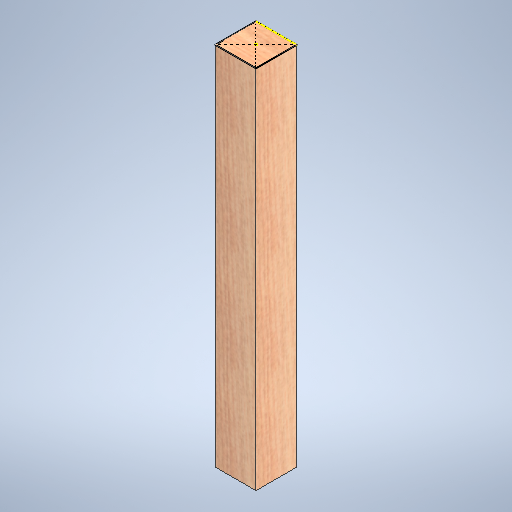
# Autodesk Inventor part: 4x4x36
Saved by Autodesk Inventor 2025 (Build 290162000, 162)
## iProperties
Created: 2024-06-05
Part Number: 4x4x36
Material: Wood (Birch)
Document SubType Name: Modeling
Designer: Cupri
Density: 0.55 g/cm^3
Appearance: Birch - Natural Polished
Author: Cupri
Autodesk Inventor part; units mm, degrees
ref_plane "YZ Plane" through (0, 0, 0) normal (1, 0, 0) x (0, 1, 0)
ref_plane "XZ Plane" through (0, 0, 0) normal (0, 1, 0) x (-1, 0, 0)
ref_plane "XY Plane" through (0, 0, 0) normal (0, 0, 1) x (1, 0, 0)
sketch "Sketch1" plane through (0, 0, 0) normal (0, 1, 0) x (-1, 0, 0)
  line L0 (-50.8, 50.8) -> (-50.8, -50.8)
  line L1 (-50.8, -50.8) -> (50.8, -50.8)
  line L2 (50.8, -50.8) -> (50.8, 50.8)
  line L3 (50.8, 50.8) -> (-50.8, 50.8)
  line L4 (-50.8, 50.8) -> (50.8, -50.8) construction
  line L5 (-50.8, -50.8) -> (50.8, 50.8) construction
  point P0 (0, 0)
  dimension "d0" = 101.6
  dimension "d1" = 101.6
  constraints: 12 end point, 2 midpoint, 2 parallel, 1 perpendicular, 1 vertical
  measures "d0" distance of L0.start L0.end
  measures "d1" distance of L1.end L0.end
extrude "Extrusion1" add sketch "Sketch1" along normal blind 914.4
sketch "Sketch2" plane through (0, 914.4, 0) normal (0, 1, 0) x (1, 0, 0)
  line L0 (50.8, 50.8) -> (-50.8, 50.8) projected
  line L1 (50.8, -50.8) -> (-50.8, -50.8)
  line L2 (-50.8, -50.8) -> (-50.8, 50.8)
  line L3 (-50.8, 50.8) -> (50.8, 50.8)
  line L4 (50.8, 50.8) -> (50.8, -50.8)
  line L5 (50.8, -50.8) -> (-50.8, 50.8) construction
  line L6 (-50.8, -50.8) -> (50.8, 50.8) construction
  point P0 (0, 0)
  constraints: 12 end point, 2 midpoint, 2 parallel, 1 horizontal, 1 perpendicular
body "Solid1"
